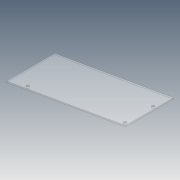
# Autodesk Inventor part: GE-12087-03
Saved by Autodesk Inventor 2012 (Build 160160000, 160)
## iProperties
Created: 2011-10-10
Part Number: GE-12087-03
Document SubType Name: Modeling
Designer: dfoster
Density: 1 g/cm^3
Description: Top
Material: Default
Title: Top
Author: dfoster
Autodesk Inventor part; units mm, degrees
ref_plane "YZ Plane" through (0, 0, 0) normal (1, 0, 0) x (0, 1, 0)
ref_plane "XZ Plane" through (0, 0, 0) normal (0, 1, 0) x (-1, 0, 0)
ref_plane "XY Plane" through (0, 0, 0) normal (0, 0, 1) x (1, 0, 0)
sketch "Sketch1" plane through (0, 0, 0) normal (0, 0, 1) x (1, 0, 0)
  line L0 (-157.9563, -24.9852) -> (132.5562, 26.24) projected
  line L1 (132.5562, 29.4639) -> (132.5562, 26.24) projected
  line L2 (132.5562, 29.4639) -> (-157.9563, -21.7613) projected
  line L3 (-157.9563, -24.9852) -> (-157.9563, -21.7613) projected
  point P0 (0, 0)
extrude "Extrusion1" add sketch "Sketch1" along normal blind 117.475
hole "Hole1" at (123.176, 27.8099, 109.5375) direction (0.1736482, -0.9848078, 0) diameter 6.731 depth 25.4 tip angle 118
pattern_linear "Rectangular Pattern1" count 2 spacing 241.3 along (-0.9848078, -0.1736482, 0) of "Hole1"
pattern_linear "Rectangular Pattern2" count 2 spacing 68.2625 along (0, 0, -1) of "Hole1"
body "Solid1"
